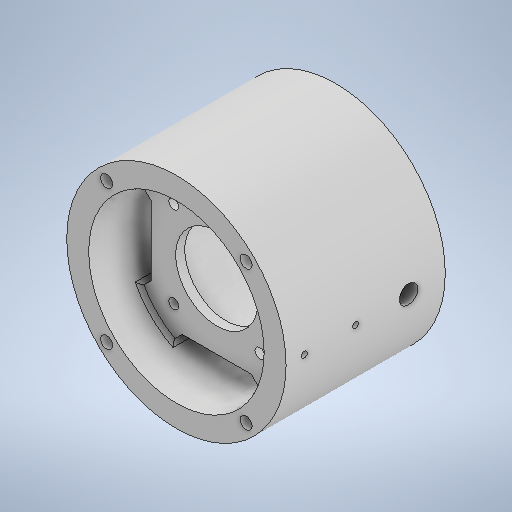
# Autodesk Inventor part: j1 57 mount
Saved by Autodesk Inventor 2025 (Build 290162000, 162)
## iProperties
Created: 2025-07-04
Part Number: j1 57 mount
Material: 一般
Document SubType Name: Modeling
Designer: gavin
Density: 1 g/cm^3
Appearance: 預設
Author: gavin
## iProperties of the stored document j1 57 mount_3D 列印.ipt
Created: 2025-07-09
Part Number: j1 57 mount_3D 列印
Material: 一般
Document SubType Name: Modeling
Designer: gavin
Density: 1 g/cm^3
Appearance: 預設
Author: gavin
Autodesk Inventor part; units mm, degrees
sketch "草圖1" plane through (0, 0, 0) normal (0, 0, 1) x (1, 0, 0)
  circle A0 centre (0, 0) radius 60
  circle A1 centre (0, 0) radius 48
  dimension "d0" = 120
  dimension "d1" = 96
  constraints: 2 centre point, 2 coincident
  measures "d0" diameter of A0
  measures "d1" diameter of A1
extrude "擠出1" add sketch "草圖1" along normal blind 27.1 and the other way blind 60
sketch "草圖2" plane through (0, 0, 27.1) normal (0, 0, 1) x (1, 0, 0)
  circle A0 centre (0, 0) radius 54 construction
  circle A1 centre (38.183766, 38.183766) radius 3.275
  circle A2 centre (-38.183766, 38.183766) radius 3.275
  circle A3 centre (-38.183766, -38.183766) radius 3.275
  circle A4 centre (38.183766, -38.183766) radius 3.275
  line L0 (0, 0) -> (-38.183766, -38.183766) construction
  line L1 (0, 0) -> (54, 0) construction
  dimension "d6" = 108
  dimension "d7" = 6.55
  dimension "d10" = 360
  dimension "d62" = 135
  constraints: 5 centre point, 4 end point, 2 coincident, 2 point on circle, 1 equal length, 1 horizontal, 9 other
  measures "d6" diameter of A0
  measures "d7" diameter of A1
  measures "d62" angle of L0 L1
extrude "擠出2" cut sketch "草圖2" against normal blind 20
ref_plane "工作平面1" through (0, 0, 0) normal (0, 0, 1) x (1, 0, 0)
sketch "草圖3" plane through (0, 0, 0) normal (0, 0, 1) x (1, 0, 0)
  circle A0 centre (-23.57, 23.57) radius 2.3
  circle A1 centre (23.57, 23.57) radius 2.3
  circle A2 centre (23.57, -23.57) radius 2.3
  circle A3 centre (-23.57, -23.57) radius 2.3
  circle A4 centre (-23.57, 23.57) radius 2.7
  circle A5 centre (23.57, 23.57) radius 2.7
  circle A6 centre (23.57, -23.57) radius 2.7
  circle A7 centre (-23.57, -23.57) radius 2.7
  circle A8 centre (0, 0) radius 22.5
  line L0 (-21.94355, 4.972987) -> (-41.348635, 24.378072)
  circle A9 centre (0, 0) radius 48
  line L1 (-24.378072, 41.348635) -> (-4.972987, 21.94355)
  line L2 (-23.57, 23.57) -> (0, 0) construction
  circle A10 centre (0, 0) radius 40.5
  line L3 (-41.348635, -24.378072) -> (-21.94355, -4.972987)
  line L4 (-4.972987, -21.94355) -> (-24.378072, -41.348635)
  line L5 (24.378072, -41.348635) -> (4.972987, -21.94355)
  line L6 (21.94355, -4.972987) -> (41.348635, -24.378072)
  line L7 (41.348635, 24.378072) -> (21.94355, 4.972987)
  line L8 (4.972987, 21.94355) -> (24.378072, 41.348635)
  point P0 (-18.866592, 35.837155)
  point P1 (-35.837155, 18.866592)
  point P2 (-35.837155, -18.866592)
  point P3 (-24.378072, -41.348635)
  point P4 (-18.866592, -35.837155)
  point P5 (18.866592, -35.837155)
  point P6 (24.378072, -41.348635)
  point P7 (41.348635, -24.378072)
  point P8 (35.837155, -18.866592)
  point P9 (35.837155, 18.866592)
  point P10 (41.348635, 24.378072)
  point P11 (24.378072, 41.348635)
  point P12 (18.866592, 35.837155)
  dimension "d14" = 5.4
  dimension "d15" = 5.4
  dimension "d16" = 5.4
  dimension "d17" = 5.4
  dimension "d18" = 45
  dimension "d19" = 24
  dimension "d20" = 12
  dimension "d21" = 18
  dimension "d24" = 360
  constraints: 18 end point, 6 centre point, 4 point on circle, 2 coincident, 2 parallel, 25 other
  measures "d14" diameter of A4
  measures "d15" diameter of A5
  measures "d16" diameter of A6
  measures "d17" diameter of A7
  measures "d18" diameter of A8
  measures "d19" distance between parallel lines of L1 L0
  measures "d20" distance from line of A0.centre L1
  measures "d21" radial gap between concentric circles of A8 A10
extrude "擠出3" add sketch "草圖3" along normal blind 5 contours A8 L7 A10 L6 | A8 L8 A10 L7 | L6 A10 L5 A8 | A8 L1 A10 L8 | A10 L8 A9 L7 | L5 A10 L4 A8 | L6 A9 L5 A10 | A8 L0 A10 L1 | L4 A10 L3 A8 | A8 L3 A10 L0 | A10 L0 A9 L1 | L4 A9 L3 A10
fillet "圓角1" radius 2 16 edges at (-33.9411, 33.9411, 5) (-41.3486, 24.3781, 2.5) (33.9411, 33.9411, 5) (41.3486, 24.3781, 2.5) (41.3486, -24.3781, 2.5) (33.9411, -33.9411, 5) (-33.9411, -33.9411, 5) (-41.3486, -24.3781, 2.5) (24.3781, 41.3486, 2.5) (24.3781, -41.3486, 2.5) (-24.3781, 41.3486, 2.5) (-24.3781, -41.3486, 2.5) (33.9411, -33.9411, 0) (-33.9411, -33.9411, 0) (-33.9411, 33.9411, 0) (33.9411, 33.9411, 0)
sketch "草圖4" plane through (0, 0, -60) normal (0, 0, -1) x (-1, 0, 0)
  circle A0 centre (0, 0) radius 54 construction
  line L0 (0, 0) -> (46.765372, 27) construction
  line L1 (0, 0) -> (54, 0) construction
  circle A1 centre (46.765372, 27) radius 3.275
  line L2 (0, 0) -> (0, 54) construction
  circle A2 centre (0, 54) radius 3.275
  line L3 (0, 0) -> (-46.765372, 27) construction
  circle A3 centre (-46.765372, 27) radius 3.275
  line L4 (0, 0) -> (-46.765372, -27) construction
  circle A4 centre (-46.765372, -27) radius 3.275
  line L5 (0, 0) -> (0, -54) construction
  circle A5 centre (0, -54) radius 3.275
  line L6 (0, 0) -> (46.765372, -27) construction
  circle A6 centre (46.765372, -27) radius 3.275
  dimension "d65" = 108
  dimension "d66" = 30
  dimension "d67" = 6.55
  dimension "d70" = 360
  constraints: 14 end point, 8 coincident, 6 centre point, 1 equal length, 1 horizontal, 32 other
  measures "d66" angle of L1 L0
  measures "d67" diameter of A1
extrude "擠出4" cut sketch "草圖4" against normal blind 20
ref_plane "工作平面2" through (28.2, -16.65, -54) normal (1, 0, 0) x (0, 1, 0)
sketch "草圖5" plane through (28.2, -16.65, -54) normal (1, 0, 0) x (0, 1, 0)
  circle A0 centre (16.65, 14) radius 5
  line L0 (-43.35, -6) -> (76.65, -6) projected
  point P0 (16.65, 54)
  dimension "d36" = 10
  dimension "d37" = 20
  constraints: 1 centre point
  measures "d36" diameter of A0
  measures "d37" distance from line of L0 A0.centre
extrude "擠出5" cut sketch "草圖5" along normal through all
sketch "草圖9" plane through (0, 0, 5) normal (0, 0, 1) x (1, 0, 0)
  arc A0 (-39.928224, -22.841561) -> (-22.841561, -39.928224) centre (0, 0) ccw
  arc A1 (-22.498585, -39.469148) -> (-22.841561, -39.928224) centre (-21.084372, -40.883362) ccw
  line L0 (-22.498585, -39.469148) -> (-18.866592, -35.837155)
  arc A2 (-18.866592, -35.837155) -> (18.866592, -35.837155) centre (0, 0) ccw
  line L1 (18.866592, -35.837155) -> (22.498585, -39.469148)
  arc A3 (22.841561, -39.928224) -> (22.498585, -39.469148) centre (21.084372, -40.883362) ccw
  arc A4 (22.841561, -39.928224) -> (39.928224, -22.841561) centre (0, 0) ccw
  arc A5 (39.469148, -22.498585) -> (39.928224, -22.841561) centre (40.883362, -21.084372) ccw
  line L2 (39.469148, -22.498585) -> (35.837155, -18.866592)
  arc A6 (35.837155, -18.866592) -> (35.837155, 18.866592) centre (0, 0) ccw
  line L3 (35.837155, 18.866592) -> (39.469148, 22.498585)
  arc A7 (39.928224, 22.841561) -> (39.469148, 22.498585) centre (40.883362, 21.084372) ccw
  arc A8 (39.928224, 22.841561) -> (22.841561, 39.928224) centre (0, 0) ccw
  arc A9 (22.498585, 39.469148) -> (22.841561, 39.928224) centre (21.084372, 40.883362) ccw
  line L4 (22.498585, 39.469148) -> (18.866592, 35.837155)
  arc A10 (18.866592, 35.837155) -> (-18.866592, 35.837155) centre (0, 0) ccw
  line L5 (-18.866592, 35.837155) -> (-22.498585, 39.469148)
  arc A11 (-22.841561, 39.928224) -> (-22.498585, 39.469148) centre (-21.084372, 40.883362) ccw
  arc A12 (-22.841561, 39.928224) -> (-39.928224, 22.841561) centre (0, 0) ccw
  arc A13 (-39.469148, 22.498585) -> (-39.928224, 22.841561) centre (-40.883362, 21.084372) ccw
  line L6 (-39.469148, 22.498585) -> (-35.837155, 18.866592)
  arc A14 (-35.837155, 18.866592) -> (-35.837155, -18.866592) centre (0, 0) ccw
  line L7 (-35.837155, -18.866592) -> (-39.469148, -22.498585)
  arc A15 (-39.928224, -22.841561) -> (-39.469148, -22.498585) centre (-40.883362, -21.084372) ccw
  circle A16 centre (23.57, -23.57) radius 2.7
  circle A17 centre (23.57, 23.57) radius 2.7
  circle A18 centre (-23.57, 23.57) radius 2.7
  circle A19 centre (-23.57, -23.57) radius 2.7
  circle A20 centre (0, 0) radius 22.5
  line L8 (18.866592, -35.837155) -> (-18.866592, -35.837155)
  line L9 (35.837155, 18.866592) -> (35.837155, -18.866592)
  line L10 (-18.866592, 35.837155) -> (18.866592, 35.837155)
  line L11 (-35.837155, -18.866592) -> (-35.837155, 18.866592)
  point P0 (35.837155, 18.866592)
  point P1 (-18.866592, 35.837155)
  point P2 (-35.837155, -18.866592)
  dimension "d58" = 360
  constraints: 8 end point, 1 horizontal, 13 other
extrude "擠出8" cut sketch "草圖9" against normal up to surface (5 mm away) contours A14 L11 | L8 A2 | A10 L10 | L9 A6
ref_plane "工作平面4" through (48, 0, 0) normal (1, 0, 0) x (0, 1, 0)
sketch "草圖10" plane through (48, 0, 0) normal (1, 0, 0) x (0, 1, 0)
  circle A0 centre (0, 17.1) radius 1.6
  circle A1 centre (0, -10.9) radius 1.6
  line L0 (-48, 27.1) -> (48, 27.1) projected
  circle A2 centre (0, -10.9) radius 3.1
  circle A3 centre (0, 17.1) radius 3.1
  point P0 (0, 0)
  point P1 (0, 27.1)
  dimension "d73" = 3.2
  dimension "d74" = 3.2
  dimension "d75" = 10
  dimension "d76" = 28
  dimension "d77" = 1.5
  dimension "d78" = 1.5
  constraints: 4 centre point, 1 midpoint
  measures "d73" diameter of A0
  measures "d74" diameter of A1
  measures "d75" distance of point (0, 27.1) A0.centre
  measures "d76" distance of A1.centre A0.centre
  measures "d77" radial gap between concentric circles of A1 A2
  measures "d78" radial gap between concentric circles of A0 A3
extrude "擠出9" add sketch "草圖10" against normal blind 1
fillet "圓角2" radius 1 6 edges at (47.8998, -3.1, 17.0969) (47.9421, 2.3576, 19.1128) (47.942, 2.3586, 15.0883) (47.8998, -3.1, -10.9031) (47.942, 2.3586, -12.9117) (47.9421, 2.3576, -8.8872)
sketch "草圖11" plane through (47, 0, 17.1) normal (-1, 0, 0) x (0, 0, 1)
  circle A0 centre (0, 0) radius 1.6 projected
  circle A1 centre (-28, 0) radius 1.6 projected
  point P0 (-17.1, 0)
extrude "擠出10" cut sketch "草圖11" against normal through all
sketch "草圖12" plane through (0, 0, 5) normal (0, 0, 1) x (1, 0, 0)
  line L0 (35.837155, -18.866592) -> (35.837155, 18.866592)
  line L1 (35.837155, 6.866592) -> (32.837155, 6.866592)
  line L2 (27.837155, 1.866592) -> (27.837155, -1.866592)
  line L3 (32.837155, -6.866592) -> (35.837155, -6.866592)
  line L4 (35.837155, -6.866592) -> (35.837155, 6.866592)
  arc A0 (32.837155, 6.866592) -> (27.837155, 1.866592) centre (32.837155, 1.866592) ccw
  arc A1 (27.837155, -1.866592) -> (32.837155, -6.866592) centre (32.837155, -1.866592) ccw
  point P0 (0, 0)
  point P1 (27.837155, 6.866592)
  dimension "d84" = 12
  dimension "d85" = 12
  dimension "d86" = 8
  dimension "d87" = 5
  constraints: 8 end point, 4 point on circle, 4 tangent, 3 point on line, 2 centre point, 2 parallel, 1 equal radius, 1 horizontal, 1 perpendicular
  measures "d84" distance from line of L0.end L1
  measures "d85" distance from line of L3 L0.start
  measures "d86" distance of L1.start point (27.837, 6.867)
  measures "d87" radius of A0
extrude "擠出11" cut sketch "草圖12" against normal through all
fillet "圓角3" radius 5 2 edges at (35.8372, -6.8666, 2.5) (35.8372, 6.8666, 2.5)
equation "\"d20\" = 0.5 * d19"
equation "\"d85\" = d84"
